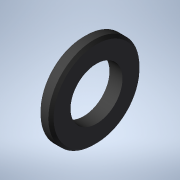
# Autodesk Inventor part: CLBU4-7-1
Saved by Autodesk Inventor 2021 (Build 250183000, 183)
## iProperties
Created: 2025-03-05
Part Number: CLBU4-7-1
Material: Generic
Catalog Web Link: www.cadenas.de
Description: CLBU, CLBUB, CLBUM, CLBUS,  CLBP, CLBPB, CLBPM, CLBPS-Bearing Spacers - For Inner Ring
Vendor: MISUMI
Document SubType Name: Modeling
Designer: psAdmin
Manufacturer: MISUMI
Mass: 0.0250552 g
Surface Area: 0.811368 cm^2
Volume: 0.0250552 cm^3
Density: 1 g/cm^3
Appearance: PSOLRGB-191-191-191
Category: PARTsolutions
Company: MISUMI
Title: CLBU4-7-1
Author: Cadenas PARTsolutions
Comments: Bearing Spacers - For Inner Ring
PSOL_IDENT_0: {$CADENAS_DATA/23d-libs/misumi/metric/12_bearing_holders/clbu.prj},230 {VTYP=3D},{NB=CLBU4-7-1},{LIN
PSOL_IDENT_1: A=CLBU4-7-1},{NN=CLBU, CLBUB, CLBUM, CLBUS,  CLBP, CLBPB, CLBPM, CLBPS},{DATE=09.09.2019 15:26:56},{
PSOL_IDENT_2: GEOMDATE=08.10.2015 00:14:34},{VERSION=},{LINEID=20},{WBVAR=LTOL,MAT,ST,DD,L,ALT1},{WBNUMERIC=DD,L}
PSOL_IDENT_3: {NB=CLBU4-7-1},{LINA=CLBU4-7-1},{KT=DUMMY},{PN=CLBU4-7-1},{TYPE=CLBU},{TS11=3},{LTOL=M},{MAT=},{MAT
PSOL_IDENT_4: ALG= '', 'Aluminum Alloy 5000 series', 'BM', 'Low Carbon Steel', 'S' , 'SUS304' },{ST=},{ST1=   '','
PSOL_IDENT_5: -'         },{D=7},{D1=7},{DD=4},{L=1.0},{L1= [1.0:50.0/0.1]},{ALT1=},{ALT1ALG='','w/o LKC (Overall
PSOL_IDENT_6: Length Tolerance)','-LKC','with LKC (Overall Length Tolerance)'},{LTOL1=0/-0.1},{DSS=6},{DD1=4},{AP=
PSOL_IDENT_7: 674ZZ,694ZZ,624ZZ},{LTEMP=.0},{DPN=7},{DSSPN=CLBU47-1},{ALT1PN=},{DDPN=4},{COLOR=0.75,0.75,0.75,0.00
PSOL_IDENT_8: }
NB: CLBU4-7-1
NN: CLBU, CLBUB, CLBUM, CLBUS,  CLBP, CLBPB, CLBPM, CLBPS
NT: Bearing Spacers - For Inner Ring
NBSYN: $PN.
LINA: CLBU4-7-1
CATALOG: Misumi
PN: CLBU4-7-1
LTOL: Negative Tolerance
MAT: Aluminum Alloy 5000 series
ST: -
D: 7
DD: 4
L: 1
ALT1: w/o LKC (Overall Length Tolerance)
DSS: 6
AP: 674ZZ,694ZZ,624ZZ
SUPPLIER: MISUMI
ARTICLENO: CLBU4-7-1
BOMINFO: CLBU4-7-1
CREATOR: CADENAS GmbH
Autodesk Inventor part; units mm, degrees
sketch "Sketch_1" plane through (0, 0, 0) normal (0, 0, 1) x (1, 0, 0)
  line L0 (1, 0) -> (0, 0)
  line L1 (0, 2) -> (1, 2)
  line L2 (1, 2) -> (1, 3.3)
  line L3 (1, 3.3) -> (0.8, 3.5)
  line L4 (0.8, 3.5) -> (0.2, 3.5)
  line L5 (0.2, 3.5) -> (0, 3.3)
  line L6 (0, 3.3) -> (0, 2)
  constraints: 14 end point
revolve "Revolution1" add sketch "Sketch_1" angle 360 about axis through (1, 0, 0) along (1, 0, 0)
ref_plane "to_b_XY" through (0, 0, 0) normal (1, 0, 0) x (0, 0, -1)
ref_plane "to_b_YZ" through (0, 0, 0) normal (0, 0, -1) x (0, 1, 0)
ref_plane "to_b_ZX" through (0, 0, 0) normal (0, 1, 0) x (1, 0, 0)
body "Solid1"
